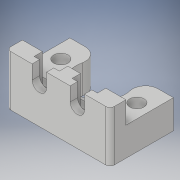
# Autodesk Inventor part: bltouch_mount_aio_base
Saved by Autodesk Inventor 2019.4 (Build 234330000, 330)
## iProperties
Created: 2020-09-18
Part Number: bltouch_mount_aio_base
Material: Generisch
Document SubType Name: Modeling
Designer: marc
Density: 1 g/cm^3
Appearance: Vorgabe
Author: marc
## iProperties of the stored document _3D-Druck.ipt
Created: 2020-10-24
Part Number: _3D-Druck
Material: Generisch
Document SubType Name: Modeling
Designer: marc
Density: 1 g/cm^3
Appearance: Vorgabe
Author: marc
Autodesk Inventor part; units mm, degrees
ref_plane "YZ Plane" through (0, 0, 0) normal (1, 0, 0) x (0, 1, 0)
ref_plane "XZ Plane" through (0, 0, 0) normal (0, 1, 0) x (-1, 0, 0)
ref_plane "XY Plane" through (0, 0, 0) normal (0, 0, 1) x (1, 0, 0)
sketch "Skizze1" plane through (0, 0, 0) normal (0, 0, 1) x (1, 0, 0)
  line L0 (0, 0) -> (-24.5, 0)
  line L1 (-24.5, 0) -> (-24.5, 7)
  line L2 (-24.5, 7) -> (0, 7)
  line L3 (0, 7) -> (0, 0)
  dimension "d0" = 24.5
  dimension "d1" = 7
  constraints: 8 end point, 2 parallel, 1 horizontal, 1 perpendicular
  measures "d0" distance of L1.end L2.end
  measures "d1" distance of L2.end L0.start
extrude "Extrusion1" add sketch "Skizze1" along normal blind 18.4
sketch "Skizze2" plane through (0, 0, 18.4) normal (0, 0, 1) x (1, 0, 0)
  line L0 (0, 7) -> (-24.5, 7) projected
  line L1 (0, 0) -> (0, 7) projected
  point P0 (-21.45, 2.7)
  point P1 (-3.05, 2.7)
  dimension "d4" = 4.3
  dimension "d5" = 18.4
  dimension "d6" = 3.05
  dimension "d7" = 24.5
  constraints: 1 horizontal alignment
  measures "d4" distance from line of L0 point (-3.05, 2.7)
  measures "d5" distance of point (-3.05, 2.7) point (-21.45, 2.7)
  measures "d6" distance from line of L1 point (-3.05, 2.7)
  measures "d7" distance of L0.start L0.end
hole "Bohrung1" at (-21.45, 2.7, 18.4) at (-3.05, 2.7, 18.4) direction (0, 0, -1) diameter 4.3 depth 10 clearance for "Senkschraube mit Linsenkopf ISO 2010" size "M4" standard "DIN"
sketch "Skizze4" plane through (0, 0, 0) normal (1, 0, 0) x (0, 0, -1)
  line L0 (-18.4, 0) -> (-18.4, 7) projected
  line L1 (0, 0) -> (-18.4, 0) projected
  point P0 (-7, 10)
  dimension "d18" = 11.4
  dimension "d19" = 10
  measures "d18" distance from line of point (-7, 10) L0
  measures "d19" distance from line of L1 point (-7, 10)
hole "Bohrung2" at (0, 10, 7) direction (-1, 0, 0) diameter 15 depth 24.75
sketch "Skizze5" plane through (0, 0, 0) normal (0, 0, -1) x (-1, 0, 0)
  line L0 (0, 0) -> (24.5, 0) projected
  line L1 (0, 0) -> (24.5, 0)
  line L2 (24.5, 0) -> (24.5, 23)
  line L3 (24.5, 23) -> (0, 23)
  line L4 (0, 23) -> (0, 0)
  dimension "d27" = 23
  constraints: 8 end point, 2 parallel, 1 horizontal, 1 perpendicular
  measures "d27" distance of L0.end L2.end
extrude "Extrusion3" add sketch "Skizze5" along normal blind 3
sketch "Skizze8" plane through (0, 0, -3) normal (0, 0, -1) x (-1, 0, 0)
  line L0 (0, 16) -> (24.5, 16)
  line L1 (24.5, 16) -> (24.5, 23)
  line L2 (24.5, 23) -> (0, 23)
  line L3 (0, 23) -> (0, 16)
  line L4 (0, 23) -> (0, 0) projected
  line L5 (24.5, 0) -> (24.5, 23) projected
  line L6 (24.5, 23) -> (0, 23) projected
  dimension "d44" = 7
  constraints: 8 end point, 2 parallel, 2 point on line, 1 horizontal, 1 perpendicular
  measures "d44" distance of L1.end L0.end
extrude "Extrusion4" add sketch "Skizze8" along normal blind 12
sketch "Skizze9" plane through (-24.5, 23, -3) normal (0, 1, 0) x (1, 0, 0)
  line L0 (0, -3) -> (24.5, -3) projected
  line L1 (24.5, -3) -> (24.5, 12) projected
  line L2 (0, -3) -> (0, 12) projected
  point P0 (12.25, 7)
  dimension "d115" = 24.5
  dimension "d116" = 12.25
  dimension "d118" = 10
  measures "d115" distance of L0.start L0.end
  measures "d116" distance from line of L2 point (12.25, 7)
  measures "d118" distance from line of L0 point (12.25, 7)
hole "Bohrung4" at (-12.25, 23, -10) direction (0, -1, 0) diameter 11.7 depth 24.75
fillet "Rundung3" radius 3 2 edges at (-9.2131, 19.5, -15) (-15.2869, 19.5, -15)
sketch "Skizze6" plane through (0, 0, -3) normal (0, 0, -1) x (-1, 0, 0)
  line L0 (24.5, 23) -> (0, 23) projected
  circle A0 centre (3.05, 2.7) radius 2.15 projected
  point P0 (0, 0)
  point P1 (7.75, 19.7)
  point P2 (16.75, 19.7)
  dimension "d32" = 4.7
  dimension "d33" = 9
  dimension "d41" = 17
  constraints: 1 horizontal alignment
  measures "d32" horizontal distance of point (7.75, 19.7) A0.centre
  measures "d33" distance of point (7.75, 19.7) point (16.75, 19.7)
  measures "d41" vertical distance of A0.centre point (7.75, 19.7)
hole "Bohrung5" at (-7.75, 19.7, -3) at (-16.75, 19.7, -3) direction (0, 0, 1) diameter 3.4 depth 24.75 start extended yes clearance for "Inbusschraube DIN EN ISO 4762" size "M3" standard "DIN"
sketch "Skizze10" plane through (-24.5, 23, -3) normal (0, 1, 0) x (1, 0, 0)
  line L0 (20.871, 12) -> (24.5, 12) projected
  line L1 (0, -3) -> (0, 12) projected
  line L2 (24.5, -3) -> (24.5, 12) projected
  point P0 (3.25, 6.6)
  point P1 (21.25, 6.6)
  dimension "d66" = 18
  dimension "d69" = 5.4
  dimension "d77" = 24.5
  dimension "d78" = 3.25
  constraints: 1 horizontal alignment
  measures "d66" distance of point (3.25, 6.6) point (21.25, 6.6)
  measures "d69" distance from line of L0 point (21.25, 6.6)
  measures "d77" distance between parallel lines of L1 L2
  measures "d78" distance from line of L1 point (3.25, 6.6)
hole "Bohrung6" at (-21.25, 23, -9.6) at (-3.25, 23, -9.6) direction (0, -1, 0) diameter 3.4 depth 24.75 start extended yes
fillet "Rundung4" [suppressed]
sketch "Skizze11" plane through (-24.5, 16, -15) normal (0, -1, 0) x (1, 0, 0)
  line L0 (21.25, 2.2246) -> (18.5, 3.8123)
  line L1 (18.5, 3.8123) -> (18.5, 6.9877)
  line L2 (18.5, 6.9877) -> (21.25, 8.5754)
  line L3 (21.25, 8.5754) -> (24, 6.9877)
  line L4 (24, 6.9877) -> (24, 3.8123)
  line L5 (24, 3.8123) -> (21.25, 2.2246)
  line L6 (3.25, 2.2246) -> (0.5, 3.8123)
  line L7 (0.5, 3.8123) -> (0.5, 6.9877)
  line L8 (0.5, 6.9877) -> (3.25, 8.5754)
  line L9 (3.25, 8.5754) -> (6, 6.9877)
  line L10 (6, 6.9877) -> (6, 3.8123)
  line L11 (6, 3.8123) -> (3.25, 2.2246)
  line L12 (0, 12) -> (0, 0) projected
  line L13 (24.5, 12) -> (24.5, 0) projected
  arc A0 (19.55, 5.4) -> (19.55, 5.4) centre (21.25, 5.4) ccw projected
  arc A1 (1.55, 5.4) -> (1.55, 5.4) centre (3.25, 5.4) ccw projected
  point P0 (24.5, 15)
  point P1 (0, 5.75)
  point P2 (24.5, 5.75)
  dimension "d80" = 5.5
  dimension "d81" = 5.5
  constraints: 24 end point, 2 coincident, 2 parallel, 26 other
  measures "d80" distance between parallel lines of L4 L1
  measures "d81" distance from line of L10 L6.end
extrude "Extrusion5" cut sketch "Skizze11" along normal blind 1 and the other way blind 1 contours L0 L1 L2 L3 L4 L5 | L6 L7 L8 L9 L10 L11 | A0 | A1
sketch "Skizze12" plane through (0, 0, -3) normal (0, 0, -1) x (-1, 0, 0)
  circle A0 centre (7.75, 19.7) radius 3
  circle A1 centre (16.75, 19.7) radius 3
  circle A2 centre (16.75, 19.7) radius 1.7 projected
  circle A3 centre (7.75, 19.7) radius 1.7 projected
  point P0 (0, 0)
  dimension "d86" = 6
  dimension "d87" = 6
  constraints: 2 centre point, 2 concentric
  measures "d86" diameter of A0
  measures "d87" diameter of A1
extrude "Extrusion6" cut sketch "Skizze12" along normal mid plane 1.5
sketch "Skizze13" plane through (-24.5, 23, 0) normal (0, 1, 0) x (1, 0, 0)
  line L0 (19.75, 3.75) -> (13.75, 3.75) projected
  line L1 (13.75, 2.25) -> (19.75, 2.25) projected
  circle A0 centre (3.25, 9.6) radius 1.7 projected
  circle A1 centre (21.25, 9.6) radius 1.7 projected
  arc A2 (6.5513, 11.322) -> (3.629, 15) centre (3.629, 12) ccw projected
  line L2 (0, 15) -> (3.629, 15) projected
  line L3 (0, 0) -> (0, 15) projected
  line L4 (0, 0) -> (24.5, 0) projected
  line L5 (24.5, 0) -> (24.5, 15) projected
  line L6 (20.871, 15) -> (24.5, 15) projected
  arc A3 (20.871, 15) -> (17.9487, 11.322) centre (20.871, 12) ccw projected
  arc A4 (6.5513, 11.322) -> (17.9487, 11.322) centre (12.25, 10) ccw projected
  line L7 (10.75, 3.75) -> (4.75, 3.75) projected
  line L8 (4.75, 2.25) -> (10.75, 2.25) projected
  line L9 (19.75, 3.75) -> (19.75, 2.25)
  line L10 (13.75, 2.25) -> (13.75, 3.75)
  line L11 (10.75, 2.25) -> (10.75, 3.75)
  line L12 (4.75, 2.25) -> (4.75, 3.75)
  constraints: 8 end point, 3 parallel, 1 point on line, 1 vertical
extrude "Extrusion7" cut sketch "Skizze13" against normal blind 6.9 contours L9 L1 L10 L0 | L11 L8 L12 L7
sketch "Skizze14" plane through (0, 0, 0) normal (0, 0, 1) x (1, 0, 0)
  circle A0 centre (-7.75, 19.7) radius 1.7 projected
  line L0 (-4.75, 23) -> (-10.75, 23) projected
  line L1 (-6.05, 19.7) -> (-9.45, 19.7)
  line L2 (-9.45, 19.7) -> (-9.45, 23)
  line L3 (-9.45, 23) -> (-6.05, 23)
  line L4 (-6.05, 23) -> (-6.05, 19.7)
  line L5 (-15.05, 19.7) -> (-18.45, 19.7)
  line L6 (-18.45, 19.7) -> (-18.45, 23)
  line L7 (-18.45, 23) -> (-15.05, 23)
  line L8 (-15.05, 23) -> (-15.05, 19.7)
  circle A1 centre (-7.75, 19.7) radius 1.7 projected
  circle A2 centre (-16.75, 19.7) radius 1.7 projected
  point P0 (0, 0)
  constraints: 16 end point, 4 parallel, 3 point on circle, 3 point on line, 2 horizontal, 2 perpendicular, 1 coincident, 1 horizontal alignment, 1 midpoint, 1 other
extrude "Extrusion8" cut sketch "Skizze14" against normal blind 2.5
move faces "Verschieben1" translate (0, 0, 0.5) faces at (-16.6817, 16.7375, -2.25) (-7.8183, 16.7375, -2.25)
fillet "Rundung7" radius 1 4 edges at (-24.5, 15, 0) (-24.5, 2.5, 7) (0, 15, 0) (0, 2.5, 7)
move faces "Verschieben2" translate (0, -5, 0) faces at (-2.6667, 16, -4.1415)
move faces "Verschieben3" translate (0, -4, 0) faces at (-18.8541, 17, -9.5317) (-5.6459, 17, -9.5317)
sketch "Skizze17" plane through (-12.25, 23, -10) normal (0, 1, 0) x (1, 0, 0)
  line L0 (-12.25, -6.25) -> (12.25, -6.25)
  line L1 (12.25, -6.25) -> (12.25, 5)
  line L2 (12.25, 5) -> (-12.25, 5)
  line L3 (-12.25, 5) -> (-12.25, -6.25)
  line L4 (-12.25, -9) -> (-12.25, 5) projected
  line L5 (12.25, -9) -> (12.25, 5) projected
  point P0 (12.25, -10)
  point P1 (-7.5, -6.25)
  constraints: 8 end point, 2 parallel, 2 point on line, 1 horizontal, 1 horizontal alignment, 1 perpendicular
extrude "Extrusion9" cut sketch "Skizze17" against normal blind 5.2
sketch "Skizze18" plane through (0, 0, -3) normal (0, 0, -1) x (-1, 0, 0)
  line L0 (24.5, 11) -> (0, 11) projected
  line L1 (0, 11) -> (0, 0) projected
  line L2 (0, 0) -> (24.5, 0) projected
  line L3 (24.5, 0) -> (24.5, 11) projected
extrude "Extrusion10" cut sketch "Skizze18" against normal blind 89.45
equation "\"d6\" = -0.5 * d5 + 0.5 * d7"
equation "\"d116\" = 0.5 * d115"
equation "\"d78\" = -0.5 * d66 + 0.5 * d77"
equation "\"d81\" = d80"
equation "\"d86\" = d87"
